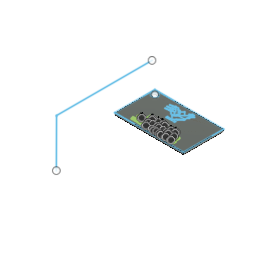
RilievoBianco_Sotto v3 (Autodesk Fusion 360 design; units mm, degrees)
Autodesk Fusion 360 part; units mm, degrees
(part 1 of 3)
sketch "Schizzo1" plane through (0, 0, 0) normal (0, 0, 1) x (1, 0, 0)
  line L0 (29.9889, 19.8901) -> (35.7373, 25.5017)
  line L1 (35.7373, 25.5017) -> (35.7373, 24.6846)
  line L2 (35.7373, 24.6846) -> (32.7498, 21.7683)
  line L3 (32.7498, 21.7683) -> (31.9129, 21.7684)
  line L4 (29.9889, 19.8901) -> (27.2751, 22.7249)
  line L5 (27.2751, 22.7249) -> (35.7303, 31.137)
  line L6 (35.7303, 31.137) -> (35.7373, 25.5017)
  line L7 (38.3163, 31.1397) -> (33.9148, 31.1342)
  line L8 (33.9148, 31.1342) -> (35.384, 32.596)
  line L9 (35.384, 32.596) -> (37.5408, 30.4282)
  line L10 (36.195, 31.7809) -> (36.8338, 32.4164)
  line L11 (36.8338, 32.4164) -> (36.8347, 31.1379)
  line L12 (38.3163, 31.1397) -> (35.7333, 28.7697)
  line L13 (36.8653, 29.8084) -> (36.8653, 28.1654)
  line L14 (36.8653, 28.1654) -> (35.7353, 27.1286)
  line L15 (32.8059, 28.2274) -> (30.0244, 31.0231)
  line L16 (30.0244, 31.0231) -> (27.8739, 28.8836)
  line L17 (27.8739, 28.8836) -> (26.8333, 29.9295)
  line L18 (26.8333, 29.9295) -> (25.5405, 29.9295)
  line L19 (25.5405, 29.9295) -> (24.3739, 31.102)
  line L20 (24.3739, 31.102) -> (22.1284, 31.102)
  line L21 (22.1284, 31.102) -> (28.8771, 24.3187)
  line L22 (28.8276, 26.6255) -> (25.5405, 29.9295)
  line L23 (-23.3316, 55.811) -> (-23.3316, -27.624)
  line L24 (-23.3316, -27.624) -> (-22.8957, -28.0621)
  line L25 (-22.8957, -28.0621) -> (18.3372, -69.5062)
  line L26 (22.1284, 31.102) -> (18.2425, 29.9166)
  line L27 (18.2425, 29.9166) -> (23.3077, 29.9166)
  line L28 (24.493, 28.7252) -> (22.0405, 28.7252)
  line L29 (22.0405, 28.7252) -> (18.2007, 27.5303)
  line L30 (18.2007, 27.5303) -> (23.0405, 27.5303)
  line L31 (23.0405, 27.5303) -> (24.0405, 26.5295)
  line L32 (24.0405, 26.5295) -> (22.5405, 26.5295)
  line L33 (22.5405, 26.5295) -> (18.724, 25.3324)
  line L34 (18.724, 25.3324) -> (23.7268, 25.3324)
  line L35 (23.7268, 25.3324) -> (25.4894, 23.6528)
  line L36 (25.4894, 23.6528) -> (28.2078, 23.6528)
  line L37 (28.2078, 23.6528) -> (25.5181, 26.5255)
  line L38 (25.5181, 26.5255) -> (24.0405, 26.5295)
  line L39 (28.8771, 24.3187) -> (27.5884, 24.3143)
  line L40 (23.0405, 27.5303) -> (22.0405, 28.7252)
  line L41 (22.5405, 26.5295) -> (23.7268, 25.3324)
  line L42 (30.085, 25.5204) -> (35.7373, 25.5017)
  line L43 (26.1075, 19.8901) -> (33.1934, 19.8901)
  line L44 (28.8276, 26.6255) -> (28.8771, 24.3187)
  line L45 (27.8739, 28.8836) -> (29.3875, 27.3623)
  line L46 (29.3875, 27.3623) -> (29.3875, 24.8264)
  line L47 (28.8566, 25.2771) -> (29.3875, 24.8264)
  line L48 (0, 34.9842) -> (60, 34.9842)
  line L49 (60, 34.9842) -> (60, -0.0158)
  line L50 (60, -0.0158) -> (0, -0.0158)
  line L51 (0, -0.0158) -> (0, 34.9842)
  line L52 (26.1075, 18.8901) -> (33.1934, 18.8901)
  line L53 (33.1934, 19.8901) -> (33.1934, 18.8901)
  line L54 (26.1075, 18.8901) -> (26.1075, 19.8901)
  line L55 (17.8462, 10.5) -> (17.8462, 13)
  line L56 (17.8462, 13) -> (18.3441, 13)
  line L57 (18.3441, 13) -> (18.9359, 11.2299)
  spline S0 degree 2 poles (18.9359, 11.2299) (19.0177, 10.9826) (19.0553, 10.8598) knots 0 0 0 1 1 1
  spline S1 degree 2 poles (19.0553, 10.8598) (19.0979, 10.9962) (19.1883, 11.2606) knots 0 0 0 1 1 1
  line L58 (19.1883, 11.2606) -> (19.7868, 13)
  line L59 (19.7868, 13) -> (20.2319, 13)
  line L60 (20.2319, 13) -> (20.2319, 10.5)
  line L61 (20.2319, 10.5) -> (19.913, 10.5)
  line L62 (19.913, 10.5) -> (19.913, 12.5924)
  line L63 (19.913, 12.5924) -> (19.1866, 10.5)
  line L64 (19.1866, 10.5) -> (18.8881, 10.5)
  line L65 (18.8881, 10.5) -> (18.1651, 12.6282)
  line L66 (18.1651, 12.6282) -> (18.1651, 10.5)
  line L67 (18.1651, 10.5) -> (17.8462, 10.5)
  spline S2 degree 2 poles (20.6122, 11.4055) (20.6122, 11.9086) (20.8919, 12.1508) knots 0 0 0 1 1 1
  spline S3 degree 2 poles (20.8919, 12.1508) (21.1255, 12.352) (21.4615, 12.352) knots 0 0 0 1 1 1
  spline S4 degree 2 poles (21.4615, 12.352) (21.8349, 12.352) (22.072, 12.1073) knots 0 0 0 1 1 1
  spline S5 degree 2 poles (22.072, 12.1073) (22.309, 11.8626) (22.309, 11.4311) knots 0 0 0 1 1 1
  spline S6 degree 2 poles (22.309, 11.4311) (22.309, 11.0815) (22.2041, 10.8811) knots 0 0 0 1 1 1
  spline S7 degree 2 poles (22.2041, 10.8811) (22.0993, 10.6808) (21.8989, 10.5699) knots 0 0 0 1 1 1
  spline S8 degree 2 poles (21.8989, 10.5699) (21.6985, 10.4591) (21.4615, 10.4591) knots 0 0 0 1 1 1
  spline S9 degree 2 poles (21.4615, 10.4591) (21.0812, 10.4591) (20.8467, 10.7029) knots 0 0 0 1 1 1
  spline S10 degree 2 poles (20.8467, 10.7029) (20.6122, 10.9468) (20.6122, 11.4055) knots 0 0 0 1 1 1
  spline S11 degree 2 poles (20.9277, 11.4055) (20.9277, 11.0576) (21.0795, 10.8845) knots 0 0 0 1 1 1
  spline S12 degree 2 poles (21.0795, 10.8845) (21.2312, 10.7115) (21.4615, 10.7115) knots 0 0 0 1 1 1
  spline S13 degree 2 poles (21.4615, 10.7115) (21.69, 10.7115) (21.8417, 10.8854) knots 0 0 0 1 1 1
  spline S14 degree 2 poles (21.8417, 10.8854) (21.9935, 11.0593) (21.9935, 11.4158) knots 0 0 0 1 1 1
  spline S15 degree 2 poles (21.9935, 11.4158) (21.9935, 11.7517) (21.8409, 11.9248) knots 0 0 0 1 1 1
  spline S16 degree 2 poles (21.8409, 11.9248) (21.6883, 12.0979) (21.4615, 12.0979) knots 0 0 0 1 1 1
  spline S17 degree 2 poles (21.4615, 12.0979) (21.2312, 12.0979) (21.0795, 11.9256) knots 0 0 0 1 1 1
  spline S18 degree 2 poles (21.0795, 11.9256) (20.9277, 11.7534) (20.9277, 11.4055) knots 0 0 0 1 1 1
  line L68 (22.6688, 10.5) -> (22.6688, 12.3111)
  line L69 (22.6688, 12.3111) -> (22.9451, 12.3111)
  line L70 (22.9451, 12.3111) -> (22.9451, 12.0535)
  spline S19 degree 2 poles (22.9451, 12.0535) (23.1446, 12.352) (23.5215, 12.352) knots 0 0 0 1 1 1
  spline S20 degree 2 poles (23.5215, 12.352) (23.6852, 12.352) (23.8225, 12.2931) knots 0 0 0 1 1 1
  spline S21 degree 2 poles (23.8225, 12.2931) (23.9598, 12.2343) (24.028, 12.1388) knots 0 0 0 1 1 1
  spline S22 degree 2 poles (24.028, 12.1388) (24.0962, 12.0433) (24.1235, 11.912) knots 0 0 0 1 1 1
  spline S23 degree 2 poles (24.1235, 11.912) (24.1405, 11.8267) (24.1405, 11.6136) knots 0 0 0 1 1 1
  line L71 (24.1405, 11.6136) -> (24.1405, 10.5)
  line L72 (24.1405, 10.5) -> (23.8336, 10.5)
  line L73 (23.8336, 10.5) -> (23.8336, 11.6016)
  spline S24 degree 2 poles (23.8336, 11.6016) (23.8336, 11.7892) (23.7977, 11.8822) knots 0 0 0 1 1 1
  spline S25 degree 2 poles (23.7977, 11.8822) (23.7619, 11.9751) (23.6707, 12.0305) knots 0 0 0 1 1 1
  spline S26 degree 2 poles (23.6707, 12.0305) (23.5795, 12.0859) (23.4567, 12.0859) knots 0 0 0 1 1 1
  spline S27 degree 2 poles (23.4567, 12.0859) (23.2606, 12.0859) (23.1182, 11.9615) knots 0 0 0 1 1 1
  spline S28 degree 2 poles (23.1182, 11.9615) (22.9758, 11.837) (22.9758, 11.4891) knots 0 0 0 1 1 1
  line L74 (22.9758, 11.4891) -> (22.9758, 10.5)
  line L75 (22.9758, 10.5) -> (22.6688, 10.5)
  line L76 (25.2814, 10.7746) -> (25.3257, 10.5034)
  spline S29 degree 2 poles (25.3257, 10.5034) (25.1961, 10.4761) (25.0938, 10.4761) knots 0 0 0 1 1 1
  spline S30 degree 2 poles (25.0938, 10.4761) (24.9267, 10.4761) (24.8346, 10.529) knots 0 0 0 1 1 1
  spline S31 degree 2 poles (24.8346, 10.529) (24.7425, 10.5819) (24.705, 10.668) knots 0 0 0 1 1 1
  spline S32 degree 2 poles (24.705, 10.668) (24.6675, 10.7541) (24.6675, 11.0304) knots 0 0 0 1 1 1
  line L77 (24.6675, 11.0304) -> (24.6675, 12.0723)
  line L78 (24.6675, 12.0723) -> (24.4424, 12.0723)
  line L79 (24.4424, 12.0723) -> (24.4424, 12.3111)
  line L80 (24.4424, 12.3111) -> (24.6675, 12.3111)
  line L81 (24.6675, 12.3111) -> (24.6675, 12.7595)
  line L82 (24.6675, 12.7595) -> (24.9727, 12.9437)
  line L83 (24.9727, 12.9437) -> (24.9727, 12.3111)
  line L84 (24.9727, 12.3111) -> (25.2814, 12.3111)
  line L85 (25.2814, 12.3111) -> (25.2814, 12.0723)
  line L86 (25.2814, 12.0723) -> (24.9727, 12.0723)
  line L87 (24.9727, 12.0723) -> (24.9727, 11.0133)
  spline S33 degree 2 poles (24.9727, 11.0133) (24.9727, 10.882) (24.9889, 10.8445) knots 0 0 0 1 1 1
  spline S34 degree 2 poles (24.9889, 10.8445) (25.0051, 10.807) (25.0418, 10.7848) knots 0 0 0 1 1 1
  spline S35 degree 2 poles (25.0418, 10.7848) (25.0784, 10.7626) (25.1467, 10.7626) knots 0 0 0 1 1 1
  spline S36 degree 2 poles (25.1467, 10.7626) (25.1978, 10.7626) (25.2814, 10.7746) knots 0 0 0 1 1 1
  line L88 (26.8213, 11.0832) -> (27.1385, 11.044)
  spline S37 degree 2 poles (27.1385, 11.044) (27.0634, 10.766) (26.8605, 10.6126) knots 0 0 0 1 1 1
  spline S38 degree 2 poles (26.8605, 10.6126) (26.6576, 10.4591) (26.3421, 10.4591) knots 0 0 0 1 1 1
  spline S39 degree 2 poles (26.3421, 10.4591) (25.9447, 10.4591) (25.712, 10.7038) knots 0 0 0 1 1 1
  spline S40 degree 2 poles (25.712, 10.7038) (25.4792, 10.9485) (25.4792, 11.3902) knots 0 0 0 1 1 1
  spline S41 degree 2 poles (25.4792, 11.3902) (25.4792, 11.8472) (25.7145, 12.0996) knots 0 0 0 1 1 1
  spline S42 degree 2 poles (25.7145, 12.0996) (25.9499, 12.352) (26.325, 12.352) knots 0 0 0 1 1 1
  spline S43 degree 2 poles (26.325, 12.352) (26.6883, 12.352) (26.9185, 12.1047) knots 0 0 0 1 1 1
  spline S44 degree 2 poles (26.9185, 12.1047) (27.1487, 11.8574) (27.1487, 11.4089) knots 0 0 0 1 1 1
  spline S45 degree 2 poles (27.1487, 11.4089) (27.1487, 11.3817) (27.147, 11.3271) knots 0 0 0 1 1 1
  line L89 (27.147, 11.3271) -> (25.7964, 11.3271)
  spline S46 degree 2 poles (25.7964, 11.3271) (25.8134, 11.0286) (25.9652, 10.8701) knots 0 0 0 1 1 1
  spline S47 degree 2 poles (25.9652, 10.8701) (26.117, 10.7115) (26.3438, 10.7115) knots 0 0 0 1 1 1
  spline S48 degree 2 poles (26.3438, 10.7115) (26.5126, 10.7115) (26.632, 10.8001) knots 0 0 0 1 1 1
  spline S49 degree 2 poles (26.632, 10.8001) (26.7514, 10.8888) (26.8213, 11.0832) knots 0 0 0 1 1 1
  line L90 (25.8134, 11.5795) -> (26.8247, 11.5795)
  spline S50 degree 2 poles (26.8247, 11.5795) (26.8042, 11.808) (26.7087, 11.9222) knots 0 0 0 1 1 1
  spline S51 degree 2 poles (26.7087, 11.9222) (26.5621, 12.0996) (26.3284, 12.0996) knots 0 0 0 1 1 1
  spline S52 degree 2 poles (26.3284, 12.0996) (26.117, 12.0996) (25.9729, 11.958) knots 0 0 0 1 1 1
  spline S53 degree 2 poles (25.9729, 11.958) (25.8288, 11.8165) (25.8134, 11.5795) knots 0 0 0 1 1 1
  line L91 (28.5334, 10.5) -> (28.5334, 13)
  line L92 (28.5334, 13) -> (29.3946, 13)
  spline S54 degree 2 poles (29.3946, 13) (29.6862, 13) (29.8397, 12.9642) knots 0 0 0 1 1 1
  spline S55 degree 2 poles (29.8397, 12.9642) (30.0546, 12.9147) (30.2063, 12.7851) knots 0 0 0 1 1 1
  spline S56 degree 2 poles (30.2063, 12.7851) (30.4042, 12.618) (30.5022, 12.3579) knots 0 0 0 1 1 1
  spline S57 degree 2 poles (30.5022, 12.3579) (30.6003, 12.0979) (30.6003, 11.7636) knots 0 0 0 1 1 1
  spline S58 degree 2 poles (30.6003, 11.7636) (30.6003, 11.4789) (30.5338, 11.2589) knots 0 0 0 1 1 1
  spline S59 degree 2 poles (30.5338, 11.2589) (30.4673, 11.0389) (30.3632, 10.8948) knots 0 0 0 1 1 1
  spline S60 degree 2 poles (30.3632, 10.8948) (30.2592, 10.7507) (30.1356, 10.668) knots 0 0 0 1 1 1
  spline S61 degree 2 poles (30.1356, 10.668) (30.0119, 10.5853) (29.8371, 10.5426) knots 0 0 0 1 1 1
  spline S62 degree 2 poles (29.8371, 10.5426) (29.6623, 10.5) (29.4355, 10.5) knots 0 0 0 1 1 1
  line L93 (29.4355, 10.5) -> (28.5334, 10.5)
  line L94 (28.8643, 10.795) -> (29.398, 10.795)
  spline S63 degree 2 poles (29.398, 10.795) (29.6453, 10.795) (29.786, 10.8411) knots 0 0 0 1 1 1
  spline S64 degree 2 poles (29.786, 10.8411) (29.9267, 10.8871) (30.0102, 10.9707) knots 0 0 0 1 1 1
  spline S65 degree 2 poles (30.0102, 10.9707) (30.1279, 11.0883) (30.1936, 11.287) knots 0 0 0 1 1 1
  spline S66 degree 2 poles (30.1936, 11.287) (30.2592, 11.4857) (30.2592, 11.7688) knots 0 0 0 1 1 1
  spline S67 degree 2 poles (30.2592, 11.7688) (30.2592, 12.161) (30.1305, 12.3716) knots 0 0 0 1 1 1
  spline S68 degree 2 poles (30.1305, 12.3716) (30.0017, 12.5822) (29.8175, 12.6538) knots 0 0 0 1 1 1
  spline S69 degree 2 poles (29.8175, 12.6538) (29.6845, 12.705) (29.3895, 12.705) knots 0 0 0 1 1 1
  line L95 (29.3895, 12.705) -> (28.8643, 12.705)
  line L96 (28.8643, 12.705) -> (28.8643, 10.795)
  line L97 (32.2561, 11.0832) -> (32.5733, 11.044)
  spline S70 degree 2 poles (32.5733, 11.044) (32.4983, 10.766) (32.2954, 10.6126) knots 0 0 0 1 1 1
  spline S71 degree 2 poles (32.2954, 10.6126) (32.0924, 10.4591) (31.7769, 10.4591) knots 0 0 0 1 1 1
  spline S72 degree 2 poles (31.7769, 10.4591) (31.3796, 10.4591) (31.1468, 10.7038) knots 0 0 0 1 1 1
  spline S73 degree 2 poles (31.1468, 10.7038) (30.9141, 10.9485) (30.9141, 11.3902) knots 0 0 0 1 1 1
  spline S74 degree 2 poles (30.9141, 11.3902) (30.9141, 11.8472) (31.1494, 12.0996) knots 0 0 0 1 1 1
  spline S75 degree 2 poles (31.1494, 12.0996) (31.3847, 12.352) (31.7599, 12.352) knots 0 0 0 1 1 1
  spline S76 degree 2 poles (31.7599, 12.352) (32.1231, 12.352) (32.3533, 12.1047) knots 0 0 0 1 1 1
  spline S77 degree 2 poles (32.3533, 12.1047) (32.5836, 11.8574) (32.5836, 11.4089) knots 0 0 0 1 1 1
  spline S78 degree 2 poles (32.5836, 11.4089) (32.5836, 11.3817) (32.5819, 11.3271) knots 0 0 0 1 1 1
  line L98 (32.5819, 11.3271) -> (31.2312, 11.3271)
  spline S79 degree 2 poles (31.2312, 11.3271) (31.2483, 11.0286) (31.4001, 10.8701) knots 0 0 0 1 1 1
  spline S80 degree 2 poles (31.4001, 10.8701) (31.5518, 10.7115) (31.7786, 10.7115) knots 0 0 0 1 1 1
  spline S81 degree 2 poles (31.7786, 10.7115) (31.9475, 10.7115) (32.0668, 10.8001) knots 0 0 0 1 1 1
  spline S82 degree 2 poles (32.0668, 10.8001) (32.1862, 10.8888) (32.2561, 11.0832) knots 0 0 0 1 1 1
  line L99 (31.2483, 11.5795) -> (32.2595, 11.5795)
  spline S83 degree 2 poles (32.2595, 11.5795) (32.2391, 11.808) (32.1436, 11.9222) knots 0 0 0 1 1 1
  spline S84 degree 2 poles (32.1436, 11.9222) (31.9969, 12.0996) (31.7633, 12.0996) knots 0 0 0 1 1 1
  spline S85 degree 2 poles (31.7633, 12.0996) (31.5518, 12.0996) (31.4077, 11.958) knots 0 0 0 1 1 1
  spline S86 degree 2 poles (31.4077, 11.958) (31.2636, 11.8165) (31.2483, 11.5795) knots 0 0 0 1 1 1
  line L100 (32.9519, 10.5) -> (32.9519, 13)
  line L101 (32.9519, 13) -> (33.2589, 13)
  line L102 (33.2589, 13) -> (33.2589, 10.5)
  line L103 (33.2589, 10.5) -> (32.9519, 10.5)
  line L104 (35.9141, 11.4806) -> (35.9141, 11.7739)
  line L105 (35.9141, 11.7739) -> (36.9731, 11.7756)
  line L106 (36.9731, 11.7756) -> (36.9731, 10.8479)
  spline S87 degree 2 poles (36.9731, 10.8479) (36.7292, 10.6535) (36.47, 10.5554) knots 0 0 0 1 1 1
  spline S88 degree 2 poles (36.47, 10.5554) (36.2108, 10.4574) (35.9379, 10.4574) knots 0 0 0 1 1 1
  spline S89 degree 2 poles (35.9379, 10.4574) (35.5696, 10.4574) (35.2686, 10.6151) knots 0 0 0 1 1 1
  spline S90 degree 2 poles (35.2686, 10.6151) (34.9676, 10.7729) (34.8141, 11.0713) knots 0 0 0 1 1 1
  spline S91 degree 2 poles (34.8141, 11.0713) (34.6606, 11.3697) (34.6606, 11.7381) knots 0 0 0 1 1 1
  spline S92 degree 2 poles (34.6606, 11.7381) (34.6606, 12.103) (34.8133, 12.4193) knots 0 0 0 1 1 1
  spline S93 degree 2 poles (34.8133, 12.4193) (34.9659, 12.7357) (35.2524, 12.8892) knots 0 0 0 1 1 1
  spline S94 degree 2 poles (35.2524, 12.8892) (35.5389, 13.0426) (35.9123, 13.0426) knots 0 0 0 1 1 1
  spline S95 degree 2 poles (35.9123, 13.0426) (36.1835, 13.0426) (36.4026, 12.9548) knots 0 0 0 1 1 1
  spline S96 degree 2 poles (36.4026, 12.9548) (36.6218, 12.867) (36.7462, 12.7101) knots 0 0 0 1 1 1
  spline S97 degree 2 poles (36.7462, 12.7101) (36.8707, 12.5532) (36.9355, 12.3008) knots 0 0 0 1 1 1
  line L107 (36.9355, 12.3008) -> (36.6371, 12.219)
  spline S98 degree 2 poles (36.6371, 12.219) (36.5808, 12.41) (36.4973, 12.5191) knots 0 0 0 1 1 1
  spline S99 degree 2 poles (36.4973, 12.5191) (36.4137, 12.6282) (36.2585, 12.6939) knots 0 0 0 1 1 1
  spline S100 degree 2 poles (36.2585, 12.6939) (36.1033, 12.7595) (35.9141, 12.7595) knots 0 0 0 1 1 1
  spline S101 degree 2 poles (35.9141, 12.7595) (35.6872, 12.7595) (35.5218, 12.6905) knots 0 0 0 1 1 1
  spline S102 degree 2 poles (35.5218, 12.6905) (35.3564, 12.6214) (35.2549, 12.5089) knots 0 0 0 1 1 1
  spline S103 degree 2 poles (35.2549, 12.5089) (35.1535, 12.3963) (35.0972, 12.2616) knots 0 0 0 1 1 1
  spline S104 degree 2 poles (35.0972, 12.2616) (35.0017, 12.0297) (35.0017, 11.7585) knots 0 0 0 1 1 1
  spline S105 degree 2 poles (35.0017, 11.7585) (35.0017, 11.4243) (35.1168, 11.1992) knots 0 0 0 1 1 1
  spline S106 degree 2 poles (35.1168, 11.1992) (35.2319, 10.9741) (35.4519, 10.8649) knots 0 0 0 1 1 1
  spline S107 degree 2 poles (35.4519, 10.8649) (35.6719, 10.7558) (35.9192, 10.7558) knots 0 0 0 1 1 1
  spline S108 degree 2 poles (35.9192, 10.7558) (36.134, 10.7558) (36.3387, 10.8385) knots 0 0 0 1 1 1
  spline S109 degree 2 poles (36.3387, 10.8385) (36.5433, 10.9212) (36.649, 11.015) knots 0 0 0 1 1 1
  line L108 (36.649, 11.015) -> (36.649, 11.4806)
  line L109 (36.649, 11.4806) -> (35.9141, 11.4806)
  spline S110 degree 2 poles (38.6033, 10.7234) (38.4328, 10.5784) (38.2751, 10.5188) knots 0 0 0 1 1 1
  spline S111 degree 2 poles (38.2751, 10.5188) (38.1173, 10.4591) (37.9366, 10.4591) knots 0 0 0 1 1 1
  spline S112 degree 2 poles (37.9366, 10.4591) (37.6381, 10.4591) (37.4778, 10.6049) knots 0 0 0 1 1 1
  spline S113 degree 2 poles (37.4778, 10.6049) (37.3175, 10.7507) (37.3175, 10.9775) knots 0 0 0 1 1 1
  spline S114 degree 2 poles (37.3175, 10.9775) (37.3175, 11.1105) (37.3781, 11.2205) knots 0 0 0 1 1 1
  spline S115 degree 2 poles (37.3781, 11.2205) (37.4386, 11.3305) (37.5367, 11.397) knots 0 0 0 1 1 1
  spline S116 degree 2 poles (37.5367, 11.397) (37.6347, 11.4635) (37.7575, 11.4976) knots 0 0 0 1 1 1
  spline S117 degree 2 poles (37.7575, 11.4976) (37.8479, 11.5215) (38.0304, 11.5437) knots 0 0 0 1 1 1
  spline S118 degree 2 poles (38.0304, 11.5437) (38.4021, 11.588) (38.5778, 11.6494) knots 0 0 0 1 1 1
  spline S119 degree 2 poles (38.5778, 11.6494) (38.5795, 11.7125) (38.5795, 11.7295) knots 0 0 0 1 1 1
  spline S120 degree 2 poles (38.5795, 11.7295) (38.5795, 11.9171) (38.4925, 11.9939) knots 0 0 0 1 1 1
  spline S121 degree 2 poles (38.4925, 11.9939) (38.3748, 12.0979) (38.1429, 12.0979) knots 0 0 0 1 1 1
  spline S122 degree 2 poles (38.1429, 12.0979) (37.9263, 12.0979) (37.8232, 12.022) knots 0 0 0 1 1 1
  spline S123 degree 2 poles (37.8232, 12.022) (37.72, 11.9461) (37.6705, 11.7534) knots 0 0 0 1 1 1
  line L110 (37.6705, 11.7534) -> (37.3704, 11.7943)
  spline S124 degree 2 poles (37.3704, 11.7943) (37.4113, 11.987) (37.5051, 12.1056) knots 0 0 0 1 1 1
  spline S125 degree 2 poles (37.5051, 12.1056) (37.5989, 12.2241) (37.7763, 12.288) knots 0 0 0 1 1 1
  spline S126 degree 2 poles (37.7763, 12.288) (37.9536, 12.352) (38.1872, 12.352) knots 0 0 0 1 1 1
  spline S127 degree 2 poles (38.1872, 12.352) (38.4192, 12.352) (38.5641, 12.2974) knots 0 0 0 1 1 1
  spline S128 degree 2 poles (38.5641, 12.2974) (38.7091, 12.2428) (38.7773, 12.1601) knots 0 0 0 1 1 1
  spline S129 degree 2 poles (38.7773, 12.1601) (38.8455, 12.0774) (38.8728, 11.9512) knots 0 0 0 1 1 1
  spline S130 degree 2 poles (38.8728, 11.9512) (38.8881, 11.8728) (38.8881, 11.6681) knots 0 0 0 1 1 1
  line L111 (38.8881, 11.6681) -> (38.8881, 11.2589)
  spline S131 degree 2 poles (38.8881, 11.2589) (38.8881, 10.8308) (38.9077, 10.7174) knots 0 0 0 1 1 1
  spline S132 degree 2 poles (38.9077, 10.7174) (38.9274, 10.604) (38.9853, 10.5) knots 0 0 0 1 1 1
  line L112 (38.9853, 10.5) -> (38.6647, 10.5)
  spline S133 degree 2 poles (38.6647, 10.5) (38.617, 10.5955) (38.6033, 10.7234) knots 0 0 0 1 1 1
  spline S134 degree 2 poles (38.5778, 11.4089) (38.4106, 11.3407) (38.0764, 11.293) knots 0 0 0 1 1 1
  spline S135 degree 2 poles (38.0764, 11.293) (37.8871, 11.2657) (37.8087, 11.2316) knots 0 0 0 1 1 1
  spline S136 degree 2 poles (37.8087, 11.2316) (37.7302, 11.1975) (37.6876, 11.1318) knots 0 0 0 1 1 1
  spline S137 degree 2 poles (37.6876, 11.1318) (37.645, 11.0662) (37.645, 10.986) knots 0 0 0 1 1 1
  spline S138 degree 2 poles (37.645, 10.986) (37.645, 10.8632) (37.7379, 10.7814) knots 0 0 0 1 1 1
  spline S139 degree 2 poles (37.7379, 10.7814) (37.8308, 10.6995) (38.0099, 10.6995) knots 0 0 0 1 1 1
  spline S140 degree 2 poles (38.0099, 10.6995) (38.1872, 10.6995) (38.3254, 10.7771) knots 0 0 0 1 1 1
  spline S141 degree 2 poles (38.3254, 10.7771) (38.4635, 10.8547) (38.5283, 10.9894) knots 0 0 0 1 1 1
  spline S142 degree 2 poles (38.5283, 10.9894) (38.5778, 11.0935) (38.5778, 11.2964) knots 0 0 0 1 1 1
  line L113 (38.5778, 11.2964) -> (38.5778, 11.4089)
  line L114 (39.3571, 10.5) -> (39.3571, 13)
  line L115 (39.3571, 13) -> (39.6641, 13)
  line L116 (39.6641, 13) -> (39.6641, 10.5)
  line L117 (39.6641, 10.5) -> (39.3571, 10.5)
  line L118 (40.133, 10.5) -> (40.133, 13)
  line L119 (40.133, 13) -> (40.44, 13)
  line L120 (40.44, 13) -> (40.44, 10.5)
  line L121 (40.44, 10.5) -> (40.133, 10.5)
  spline S143 degree 2 poles (40.8015, 11.4055) (40.8015, 11.9086) (41.0812, 12.1508) knots 0 0 0 1 1 1
  spline S144 degree 2 poles (41.0812, 12.1508) (41.3148, 12.352) (41.6507, 12.352) knots 0 0 0 1 1 1
  spline S145 degree 2 poles (41.6507, 12.352) (42.0242, 12.352) (42.2613, 12.1073) knots 0 0 0 1 1 1
  spline S146 degree 2 poles (42.2613, 12.1073) (42.4983, 11.8626) (42.4983, 11.4311) knots 0 0 0 1 1 1
  spline S147 degree 2 poles (42.4983, 11.4311) (42.4983, 11.0815) (42.3934, 10.8811) knots 0 0 0 1 1 1
  spline S148 degree 2 poles (42.3934, 10.8811) (42.2885, 10.6808) (42.0882, 10.5699) knots 0 0 0 1 1 1
  spline S149 degree 2 poles (42.0882, 10.5699) (41.8878, 10.4591) (41.6507, 10.4591) knots 0 0 0 1 1 1
  spline S150 degree 2 poles (41.6507, 10.4591) (41.2705, 10.4591) (41.036, 10.7029) knots 0 0 0 1 1 1
  spline S151 degree 2 poles (41.036, 10.7029) (40.8015, 10.9468) (40.8015, 11.4055) knots 0 0 0 1 1 1
  spline S152 degree 2 poles (41.117, 11.4055) (41.117, 11.0576) (41.2688, 10.8845) knots 0 0 0 1 1 1
  spline S153 degree 2 poles (41.2688, 10.8845) (41.4205, 10.7115) (41.6507, 10.7115) knots 0 0 0 1 1 1
  spline S154 degree 2 poles (41.6507, 10.7115) (41.8793, 10.7115) (42.031, 10.8854) knots 0 0 0 1 1 1
  spline S155 degree 2 poles (42.031, 10.8854) (42.1828, 11.0593) (42.1828, 11.4158) knots 0 0 0 1 1 1
  spline S156 degree 2 poles (42.1828, 11.4158) (42.1828, 11.7517) (42.0302, 11.9248) knots 0 0 0 1 1 1
  spline S157 degree 2 poles (42.0302, 11.9248) (41.8776, 12.0979) (41.6507, 12.0979) knots 0 0 0 1 1 1
  spline S158 degree 2 poles (41.6507, 12.0979) (41.4205, 12.0979) (41.2688, 11.9256) knots 0 0 0 1 1 1
  spline S159 degree 2 poles (41.2688, 11.9256) (41.117, 11.7534) (41.117, 11.4055) knots 0 0 0 1 1 1
  line L122 (12.5989, 7.4014) -> (12.911, 7.4287)
  spline S160 degree 2 poles (12.911, 7.4287) (12.9332, 7.2411) (13.0142, 7.1209) knots 0 0 0 1 1 1
  spline S161 degree 2 poles (13.0142, 7.1209) (13.0952, 7.0007) (13.2657, 6.9265) knots 0 0 0 1 1 1
  spline S162 degree 2 poles (13.2657, 6.9265) (13.4362, 6.8523) (13.6494, 6.8523) knots 0 0 0 1 1 1
  spline S163 degree 2 poles (13.6494, 6.8523) (13.8387, 6.8523) (13.9836, 6.9086) knots 0 0 0 1 1 1
  spline S164 degree 2 poles (13.9836, 6.9086) (14.1286, 6.9649) (14.1994, 7.0629) knots 0 0 0 1 1 1
  spline S165 degree 2 poles (14.1994, 7.0629) (14.2701, 7.161) (14.2701, 7.2769) knots 0 0 0 1 1 1
  spline S166 degree 2 poles (14.2701, 7.2769) (14.2701, 7.3946) (14.2019, 7.4824) knots 0 0 0 1 1 1
  spline S167 degree 2 poles (14.2019, 7.4824) (14.1337, 7.5703) (13.9768, 7.6299) knots 0 0 0 1 1 1
  spline S168 degree 2 poles (13.9768, 7.6299) (13.8762, 7.6692) (13.5317, 7.7519) knots 0 0 0 1 1 1
  spline S169 degree 2 poles (13.5317, 7.7519) (13.1872, 7.8346) (13.0491, 7.9079) knots 0 0 0 1 1 1
  spline S170 degree 2 poles (13.0491, 7.9079) (12.8701, 8.0017) (12.7822, 8.1407) knots 0 0 0 1 1 1
  spline S171 degree 2 poles (12.7822, 8.1407) (12.6944, 8.2797) (12.6944, 8.4519) knots 0 0 0 1 1 1
  spline S172 degree 2 poles (12.6944, 8.4519) (12.6944, 8.6412) (12.8018, 8.8058) knots 0 0 0 1 1 1
  spline S173 degree 2 poles (12.8018, 8.8058) (12.9093, 8.9703) (13.1156, 9.0556) knots 0 0 0 1 1 1
  spline S174 degree 2 poles (13.1156, 9.0556) (13.322, 9.1409) (13.5744, 9.1409) knots 0 0 0 1 1 1
  spline S175 degree 2 poles (13.5744, 9.1409) (13.8523, 9.1409) (14.0646, 9.0513) knots 0 0 0 1 1 1
  spline S176 degree 2 poles (14.0646, 9.0513) (14.2769, 8.9618) (14.3912, 8.7879) knots 0 0 0 1 1 1
  spline S177 degree 2 poles (14.3912, 8.7879) (14.5055, 8.6139) (14.514, 8.3939) knots 0 0 0 1 1 1
  line L123 (14.514, 8.3939) -> (14.1968, 8.3701)
  spline S178 degree 2 poles (14.1968, 8.3701) (14.1712, 8.6071) (14.0237, 8.7282) knots 0 0 0 1 1 1
  spline S179 degree 2 poles (14.0237, 8.7282) (13.8762, 8.8492) (13.588, 8.8492) knots 0 0 0 1 1 1
  spline S180 degree 2 poles (13.588, 8.8492) (13.2879, 8.8492) (13.1506, 8.7393) knots 0 0 0 1 1 1
  spline S181 degree 2 poles (13.1506, 8.7393) (13.0133, 8.6293) (13.0133, 8.4741) knots 0 0 0 1 1 1
  spline S182 degree 2 poles (13.0133, 8.4741) (13.0133, 8.3394) (13.1105, 8.2524) knots 0 0 0 1 1 1
  spline S183 degree 2 poles (13.1105, 8.2524) (13.206, 8.1654) (13.6093, 8.0742) knots 0 0 0 1 1 1
  spline S184 degree 2 poles (13.6093, 8.0742) (14.0126, 7.9829) (14.1627, 7.9147) knots 0 0 0 1 1 1
  spline S185 degree 2 poles (14.1627, 7.9147) (14.381, 7.8141) (14.485, 7.6598) knots 0 0 0 1 1 1
  spline S186 degree 2 poles (14.485, 7.6598) (14.589, 7.5055) (14.589, 7.3042) knots 0 0 0 1 1 1
  spline S187 degree 2 poles (14.589, 7.3042) (14.589, 7.1047) (14.4748, 6.9282) knots 0 0 0 1 1 1
  spline S188 degree 2 poles (14.4748, 6.9282) (14.3605, 6.7517) (14.1465, 6.6536) knots 0 0 0 1 1 1
  spline S189 degree 2 poles (14.1465, 6.6536) (13.9325, 6.5556) (13.6647, 6.5556) knots 0 0 0 1 1 1
  spline S190 degree 2 poles (13.6647, 6.5556) (13.3254, 6.5556) (13.096, 6.6545) knots 0 0 0 1 1 1
  spline S191 degree 2 poles (13.096, 6.6545) (12.8666, 6.7534) (12.7362, 6.9521) knots 0 0 0 1 1 1
  spline S192 degree 2 poles (12.7362, 6.9521) (12.6057, 7.1508) (12.5989, 7.4014) knots 0 0 0 1 1 1
  spline S193 degree 2 poles (14.8874, 7.5038) (14.8874, 8.0068) (15.1671, 8.249) knots 0 0 0 1 1 1
  spline S194 degree 2 poles (15.1671, 8.249) (15.4008, 8.4502) (15.7367, 8.4502) knots 0 0 0 1 1 1
  spline S195 degree 2 poles (15.7367, 8.4502) (16.1102, 8.4502) (16.3472, 8.2055) knots 0 0 0 1 1 1
  spline S196 degree 2 poles (16.3472, 8.2055) (16.5842, 7.9608) (16.5842, 7.5293) knots 0 0 0 1 1 1
  spline S197 degree 2 poles (16.5842, 7.5293) (16.5842, 7.1797) (16.4794, 6.9794) knots 0 0 0 1 1 1
  spline S198 degree 2 poles (16.4794, 6.9794) (16.3745, 6.779) (16.1741, 6.6681) knots 0 0 0 1 1 1
  spline S199 degree 2 poles (16.1741, 6.6681) (15.9737, 6.5573) (15.7367, 6.5573) knots 0 0 0 1 1 1
  spline S200 degree 2 poles (15.7367, 6.5573) (15.3564, 6.5573) (15.1219, 6.8012) knots 0 0 0 1 1 1
  spline S201 degree 2 poles (15.1219, 6.8012) (14.8874, 7.045) (14.8874, 7.5038) knots 0 0 0 1 1 1
  spline S202 degree 2 poles (15.2029, 7.5038) (15.2029, 7.1559) (15.3547, 6.9828) knots 0 0 0 1 1 1
  spline S203 degree 2 poles (15.3547, 6.9828) (15.5065, 6.8097) (15.7367, 6.8097) knots 0 0 0 1 1 1
  spline S204 degree 2 poles (15.7367, 6.8097) (15.9652, 6.8097) (16.117, 6.9836) knots 0 0 0 1 1 1
  spline S205 degree 2 poles (16.117, 6.9836) (16.2688, 7.1576) (16.2688, 7.514) knots 0 0 0 1 1 1
  spline S206 degree 2 poles (16.2688, 7.514) (16.2688, 7.8499) (16.1161, 8.023) knots 0 0 0 1 1 1
  spline S207 degree 2 poles (16.1161, 8.023) (15.9635, 8.1961) (15.7367, 8.1961) knots 0 0 0 1 1 1
  spline S208 degree 2 poles (15.7367, 8.1961) (15.5065, 8.1961) (15.3547, 8.0239) knots 0 0 0 1 1 1
  spline S209 degree 2 poles (15.3547, 8.0239) (15.2029, 7.8516) (15.2029, 7.5038) knots 0 0 0 1 1 1
  line L124 (17.0174, 6.5982) -> (17.0174, 8.1705)
  line L125 (17.0174, 8.1705) -> (16.7462, 8.1705)
  line L126 (16.7462, 8.1705) -> (16.7462, 8.4093)
  line L127 (16.7462, 8.4093) -> (17.0174, 8.4093)
  line L128 (17.0174, 8.4093) -> (17.0174, 8.602)
  spline S210 degree 2 poles (17.0174, 8.602) (17.0174, 8.7844) (17.0498, 8.8731) knots 0 0 0 1 1 1
  spline S211 degree 2 poles (17.0498, 8.8731) (17.0941, 8.9925) (17.2058, 9.0667) knots 0 0 0 1 1 1
  spline S212 degree 2 poles (17.2058, 9.0667) (17.3175, 9.1409) (17.5188, 9.1409) knots 0 0 0 1 1 1
  spline S213 degree 2 poles (17.5188, 9.1409) (17.6484, 9.1409) (17.8053, 9.1102) knots 0 0 0 1 1 1
  line L129 (17.8053, 9.1102) -> (17.7592, 8.8424)
  spline S214 degree 2 poles (17.7592, 8.8424) (17.6637, 8.8595) (17.5784, 8.8595) knots 0 0 0 1 1 1
  spline S215 degree 2 poles (17.5784, 8.8595) (17.4386, 8.8595) (17.3806, 8.7998) knots 0 0 0 1 1 1
  spline S216 degree 2 poles (17.3806, 8.7998) (17.3226, 8.7401) (17.3226, 8.5764) knots 0 0 0 1 1 1
  line L130 (17.3226, 8.5764) -> (17.3226, 8.4093)
  line L131 (17.3226, 8.4093) -> (17.6756, 8.4093)
  line L132 (17.6756, 8.4093) -> (17.6756, 8.1705)
  line L133 (17.6756, 8.1705) -> (17.3226, 8.1705)
  line L134 (17.3226, 8.1705) -> (17.3226, 6.5982)
  line L135 (17.3226, 6.5982) -> (17.0174, 6.5982)
  line L136 (18.5846, 6.8728) -> (18.6289, 6.6016)
  spline S217 degree 2 poles (18.6289, 6.6016) (18.4993, 6.5744) (18.397, 6.5744) knots 0 0 0 1 1 1
  spline S218 degree 2 poles (18.397, 6.5744) (18.2299, 6.5744) (18.1378, 6.6272) knots 0 0 0 1 1 1
  spline S219 degree 2 poles (18.1378, 6.6272) (18.0457, 6.6801) (18.0082, 6.7662) knots 0 0 0 1 1 1
  spline S220 degree 2 poles (18.0082, 6.7662) (17.9707, 6.8523) (17.9707, 7.1286) knots 0 0 0 1 1 1
  line L137 (17.9707, 7.1286) -> (17.9707, 8.1705)
  line L138 (17.9707, 8.1705) -> (17.7456, 8.1705)
  line L139 (17.7456, 8.1705) -> (17.7456, 8.4093)
  line L140 (17.7456, 8.4093) -> (17.9707, 8.4093)
  line L141 (17.9707, 8.4093) -> (17.9707, 8.8578)
  line L142 (17.9707, 8.8578) -> (18.2759, 9.042)
  line L143 (18.2759, 9.042) -> (18.2759, 8.4093)
  line L144 (18.2759, 8.4093) -> (18.5846, 8.4093)
  line L145 (18.5846, 8.4093) -> (18.5846, 8.1705)
  line L146 (18.5846, 8.1705) -> (18.2759, 8.1705)
  line L147 (18.2759, 8.1705) -> (18.2759, 7.1115)
  spline S221 degree 2 poles (18.2759, 7.1115) (18.2759, 6.9802) (18.2921, 6.9427) knots 0 0 0 1 1 1
  spline S222 degree 2 poles (18.2921, 6.9427) (18.3083, 6.9052) (18.345, 6.883) knots 0 0 0 1 1 1
  spline S223 degree 2 poles (18.345, 6.883) (18.3817, 6.8608) (18.4499, 6.8608) knots 0 0 0 1 1 1
  spline S224 degree 2 poles (18.4499, 6.8608) (18.501, 6.8608) (18.5846, 6.8728) knots 0 0 0 1 1 1
  line L148 (19.219, 6.5982) -> (18.6647, 8.4093)
  line L149 (18.6647, 8.4093) -> (18.9819, 8.4093)
  line L150 (18.9819, 8.4093) -> (19.2701, 7.3639)
  line L151 (19.2701, 7.3639) -> (19.3776, 6.9751)
  spline S225 degree 2 poles (19.3776, 6.9751) (19.3844, 7.0041) (19.4714, 7.3486) knots 0 0 0 1 1 1
  line L152 (19.4714, 7.3486) -> (19.7595, 8.4093)
  line L153 (19.7595, 8.4093) -> (20.075, 8.4093)
  line L154 (20.075, 8.4093) -> (20.3462, 7.3588)
  line L155 (20.3462, 7.3588) -> (20.4366, 7.0126)
  line L156 (20.4366, 7.0126) -> (20.5406, 7.3622)
  line L157 (20.5406, 7.3622) -> (20.851, 8.4093)
  line L158 (20.851, 8.4093) -> (21.1494, 8.4093)
  line L159 (21.1494, 8.4093) -> (20.5832, 6.5982)
  line L160 (20.5832, 6.5982) -> (20.2643, 6.5982)
  line L161 (20.2643, 6.5982) -> (19.9761, 7.6828)
  line L162 (19.9761, 7.6828) -> (19.9062, 7.9915)
  line L163 (19.9062, 7.9915) -> (19.5396, 6.5982)
  line L164 (19.5396, 6.5982) -> (19.219, 6.5982)
  spline S226 degree 2 poles (22.5887, 6.8216) (22.4181, 6.6767) (22.2604, 6.617) knots 0 0 0 1 1 1
  spline S227 degree 2 poles (22.2604, 6.617) (22.1027, 6.5573) (21.9219, 6.5573) knots 0 0 0 1 1 1
  spline S228 degree 2 poles (21.9219, 6.5573) (21.6235, 6.5573) (21.4632, 6.7031) knots 0 0 0 1 1 1
  spline S229 degree 2 poles (21.4632, 6.7031) (21.3029, 6.8489) (21.3029, 7.0757) knots 0 0 0 1 1 1
  spline S230 degree 2 poles (21.3029, 7.0757) (21.3029, 7.2087) (21.3634, 7.3187) knots 0 0 0 1 1 1
  spline S231 degree 2 poles (21.3634, 7.3187) (21.4239, 7.4287) (21.522, 7.4952) knots 0 0 0 1 1 1
  spline S232 degree 2 poles (21.522, 7.4952) (21.6201, 7.5617) (21.7428, 7.5958) knots 0 0 0 1 1 1
  spline S233 degree 2 poles (21.7428, 7.5958) (21.8332, 7.6197) (22.0157, 7.6419) knots 0 0 0 1 1 1
  spline S234 degree 2 poles (22.0157, 7.6419) (22.3874, 7.6862) (22.5631, 7.7476) knots 0 0 0 1 1 1
  spline S235 degree 2 poles (22.5631, 7.7476) (22.5648, 7.8107) (22.5648, 7.8278) knots 0 0 0 1 1 1
  spline S236 degree 2 poles (22.5648, 7.8278) (22.5648, 8.0153) (22.4778, 8.0921) knots 0 0 0 1 1 1
  spline S237 degree 2 poles (22.4778, 8.0921) (22.3602, 8.1961) (22.1282, 8.1961) knots 0 0 0 1 1 1
  spline S238 degree 2 poles (22.1282, 8.1961) (21.9117, 8.1961) (21.8085, 8.1202) knots 0 0 0 1 1 1
  spline S239 degree 2 poles (21.8085, 8.1202) (21.7053, 8.0443) (21.6559, 7.8516) knots 0 0 0 1 1 1
  line L165 (21.6559, 7.8516) -> (21.3557, 7.8926)
  spline S240 degree 2 poles (21.3557, 7.8926) (21.3967, 8.0853) (21.4905, 8.2038) knots 0 0 0 1 1 1
  spline S241 degree 2 poles (21.4905, 8.2038) (21.5842, 8.3223) (21.7616, 8.3863) knots 0 0 0 1 1 1
  spline S242 degree 2 poles (21.7616, 8.3863) (21.9389, 8.4502) (22.1726, 8.4502) knots 0 0 0 1 1 1
  spline S243 degree 2 poles (22.1726, 8.4502) (22.4045, 8.4502) (22.5495, 8.3956) knots 0 0 0 1 1 1
  spline S244 degree 2 poles (22.5495, 8.3956) (22.6944, 8.3411) (22.7626, 8.2584) knots 0 0 0 1 1 1
  spline S245 degree 2 poles (22.7626, 8.2584) (22.8308, 8.1756) (22.8581, 8.0495) knots 0 0 0 1 1 1
  spline S246 degree 2 poles (22.8581, 8.0495) (22.8735, 7.971) (22.8735, 7.7664) knots 0 0 0 1 1 1
  line L166 (22.8735, 7.7664) -> (22.8735, 7.3571)
  spline S247 degree 2 poles (22.8735, 7.3571) (22.8735, 6.9291) (22.8931, 6.8157) knots 0 0 0 1 1 1
  spline S248 degree 2 poles (22.8931, 6.8157) (22.9127, 6.7023) (22.9707, 6.5982) knots 0 0 0 1 1 1
  line L167 (22.9707, 6.5982) -> (22.6501, 6.5982)
  spline S249 degree 2 poles (22.6501, 6.5982) (22.6023, 6.6937) (22.5887, 6.8216) knots 0 0 0 1 1 1
  spline S250 degree 2 poles (22.5631, 7.5072) (22.396, 7.4389) (22.0617, 7.3912) knots 0 0 0 1 1 1
  spline S251 degree 2 poles (22.0617, 7.3912) (21.8724, 7.3639) (21.794, 7.3298) knots 0 0 0 1 1 1
  spline S252 degree 2 poles (21.794, 7.3298) (21.7156, 7.2957) (21.6729, 7.23) knots 0 0 0 1 1 1
  spline S253 degree 2 poles (21.6729, 7.23) (21.6303, 7.1644) (21.6303, 7.0842) knots 0 0 0 1 1 1
  spline S254 degree 2 poles (21.6303, 7.0842) (21.6303, 6.9615) (21.7232, 6.8796) knots 0 0 0 1 1 1
  spline S255 degree 2 poles (21.7232, 6.8796) (21.8162, 6.7977) (21.9952, 6.7977) knots 0 0 0 1 1 1
  spline S256 degree 2 poles (21.9952, 6.7977) (22.1726, 6.7977) (22.3107, 6.8753) knots 0 0 0 1 1 1
  spline S257 degree 2 poles (22.3107, 6.8753) (22.4488, 6.9529) (22.5136, 7.0877) knots 0 0 0 1 1 1
  spline S258 degree 2 poles (22.5136, 7.0877) (22.5631, 7.1917) (22.5631, 7.3946) knots 0 0 0 1 1 1
  line L168 (22.5631, 7.3946) -> (22.5631, 7.5072)
  line L169 (23.3458, 6.5982) -> (23.3458, 8.4093)
  line L170 (23.3458, 8.4093) -> (23.6221, 8.4093)
  line L171 (23.6221, 8.4093) -> (23.6221, 8.1347)
  spline S259 degree 2 poles (23.6221, 8.1347) (23.7278, 8.3274) (23.8174, 8.3888) knots 0 0 0 1 1 1
  spline S260 degree 2 poles (23.8174, 8.3888) (23.9069, 8.4502) (24.0143, 8.4502) knots 0 0 0 1 1 1
  spline S261 degree 2 poles (24.0143, 8.4502) (24.1695, 8.4502) (24.3298, 8.3513) knots 0 0 0 1 1 1
  line L172 (24.3298, 8.3513) -> (24.2241, 8.0665)
  spline S262 degree 2 poles (24.2241, 8.0665) (24.1115, 8.133) (23.999, 8.133) knots 0 0 0 1 1 1
  spline S263 degree 2 poles (23.999, 8.133) (23.8984, 8.133) (23.8182, 8.0725) knots 0 0 0 1 1 1
  spline S264 degree 2 poles (23.8182, 8.0725) (23.7381, 8.0119) (23.704, 7.9045) knots 0 0 0 1 1 1
  spline S265 degree 2 poles (23.704, 7.9045) (23.6528, 7.7408) (23.6528, 7.5464) knots 0 0 0 1 1 1
  line L173 (23.6528, 7.5464) -> (23.6528, 6.5982)
  line L174 (23.6528, 6.5982) -> (23.3458, 6.5982)
  line L175 (25.752, 7.1814) -> (26.0692, 7.1422)
  spline S266 degree 2 poles (26.0692, 7.1422) (25.9942, 6.8643) (25.7913, 6.7108) knots 0 0 0 1 1 1
  spline S267 degree 2 poles (25.7913, 6.7108) (25.5883, 6.5573) (25.2728, 6.5573) knots 0 0 0 1 1 1
  spline S268 degree 2 poles (25.2728, 6.5573) (24.8755, 6.5573) (24.6427, 6.802) knots 0 0 0 1 1 1
  spline S269 degree 2 poles (24.6427, 6.802) (24.41, 7.0467) (24.41, 7.4884) knots 0 0 0 1 1 1
  spline S270 degree 2 poles (24.41, 7.4884) (24.41, 7.9454) (24.6453, 8.1978) knots 0 0 0 1 1 1
  spline S271 degree 2 poles (24.6453, 8.1978) (24.8806, 8.4502) (25.2558, 8.4502) knots 0 0 0 1 1 1
  spline S272 degree 2 poles (25.2558, 8.4502) (25.619, 8.4502) (25.8492, 8.2029) knots 0 0 0 1 1 1
  spline S273 degree 2 poles (25.8492, 8.2029) (26.0795, 7.9557) (26.0795, 7.5072) knots 0 0 0 1 1 1
  spline S274 degree 2 poles (26.0795, 7.5072) (26.0795, 7.4799) (26.0778, 7.4253) knots 0 0 0 1 1 1
  line L176 (26.0778, 7.4253) -> (24.7271, 7.4253)
  spline S275 degree 2 poles (24.7271, 7.4253) (24.7442, 7.1269) (24.896, 6.9683) knots 0 0 0 1 1 1
  spline S276 degree 2 poles (24.896, 6.9683) (25.0477, 6.8097) (25.2746, 6.8097) knots 0 0 0 1 1 1
  spline S277 degree 2 poles (25.2746, 6.8097) (25.4434, 6.8097) (25.5628, 6.8984) knots 0 0 0 1 1 1
  spline S278 degree 2 poles (25.5628, 6.8984) (25.6821, 6.987) (25.752, 7.1814) knots 0 0 0 1 1 1
  line L177 (24.7442, 7.6777) -> (25.7555, 7.6777)
  spline S279 degree 2 poles (25.7555, 7.6777) (25.735, 7.9062) (25.6395, 8.0205) knots 0 0 0 1 1 1
  spline S280 degree 2 poles (25.6395, 8.0205) (25.4928, 8.1978) (25.2592, 8.1978) knots 0 0 0 1 1 1
  spline S281 degree 2 poles (25.2592, 8.1978) (25.0477, 8.1978) (24.9036, 8.0563) knots 0 0 0 1 1 1
  spline S282 degree 2 poles (24.9036, 8.0563) (24.7595, 7.9147) (24.7442, 7.6777) knots 0 0 0 1 1 1
  line L178 (27.4642, 6.5982) -> (27.4642, 9.0982)
  line L179 (27.4642, 9.0982) -> (28.3254, 9.0982)
  spline S283 degree 2 poles (28.3254, 9.0982) (28.617, 9.0982) (28.7705, 9.0624) knots 0 0 0 1 1 1
  spline S284 degree 2 poles (28.7705, 9.0624) (28.9853, 9.013) (29.1371, 8.8834) knots 0 0 0 1 1 1
  spline S285 degree 2 poles (29.1371, 8.8834) (29.3349, 8.7162) (29.433, 8.4562) knots 0 0 0 1 1 1
  spline S286 degree 2 poles (29.433, 8.4562) (29.531, 8.1961) (29.531, 7.8619) knots 0 0 0 1 1 1
  spline S287 degree 2 poles (29.531, 7.8619) (29.531, 7.5771) (29.4645, 7.3571) knots 0 0 0 1 1 1
  spline S288 degree 2 poles (29.4645, 7.3571) (29.398, 7.1371) (29.294, 6.993) knots 0 0 0 1 1 1
  spline S289 degree 2 poles (29.294, 6.993) (29.19, 6.8489) (29.0663, 6.7662) knots 0 0 0 1 1 1
  spline S290 degree 2 poles (29.0663, 6.7662) (28.9427, 6.6835) (28.7679, 6.6409) knots 0 0 0 1 1 1
  spline S291 degree 2 poles (28.7679, 6.6409) (28.5931, 6.5982) (28.3663, 6.5982) knots 0 0 0 1 1 1
  line L180 (28.3663, 6.5982) -> (27.4642, 6.5982)
  line L181 (27.795, 6.8932) -> (28.3288, 6.8932)
  spline S292 degree 2 poles (28.3288, 6.8932) (28.5761, 6.8932) (28.7167, 6.9393) knots 0 0 0 1 1 1
  spline S293 degree 2 poles (28.7167, 6.9393) (28.8574, 6.9853) (28.941, 7.0689) knots 0 0 0 1 1 1
  spline S294 degree 2 poles (28.941, 7.0689) (29.0587, 7.1866) (29.1243, 7.3852) knots 0 0 0 1 1 1
  spline S295 degree 2 poles (29.1243, 7.3852) (29.19, 7.5839) (29.19, 7.867) knots 0 0 0 1 1 1
  spline S296 degree 2 poles (29.19, 7.867) (29.19, 8.2592) (29.0612, 8.4698) knots 0 0 0 1 1 1
  spline S297 degree 2 poles (29.0612, 8.4698) (28.9325, 8.6804) (28.7483, 8.752) knots 0 0 0 1 1 1
  spline S298 degree 2 poles (28.7483, 8.752) (28.6153, 8.8032) (28.3203, 8.8032) knots 0 0 0 1 1 1
  line L182 (28.3203, 8.8032) -> (27.795, 8.8032)
  line L183 (27.795, 8.8032) -> (27.795, 6.8932)
  line L184 (31.1869, 7.1814) -> (31.5041, 7.1422)
  spline S299 degree 2 poles (31.5041, 7.1422) (31.4291, 6.8643) (31.2261, 6.7108) knots 0 0 0 1 1 1
  spline S300 degree 2 poles (31.2261, 6.7108) (31.0232, 6.5573) (30.7077, 6.5573) knots 0 0 0 1 1 1
  spline S301 degree 2 poles (30.7077, 6.5573) (30.3104, 6.5573) (30.0776, 6.802) knots 0 0 0 1 1 1
  spline S302 degree 2 poles (30.0776, 6.802) (29.8448, 7.0467) (29.8448, 7.4884) knots 0 0 0 1 1 1
  spline S303 degree 2 poles (29.8448, 7.4884) (29.8448, 7.9454) (30.0802, 8.1978) knots 0 0 0 1 1 1
  spline S304 degree 2 poles (30.0802, 8.1978) (30.3155, 8.4502) (30.6907, 8.4502) knots 0 0 0 1 1 1
  spline S305 degree 2 poles (30.6907, 8.4502) (31.0539, 8.4502) (31.2841, 8.2029) knots 0 0 0 1 1 1
  spline S306 degree 2 poles (31.2841, 8.2029) (31.5143, 7.9557) (31.5143, 7.5072) knots 0 0 0 1 1 1
  spline S307 degree 2 poles (31.5143, 7.5072) (31.5143, 7.4799) (31.5126, 7.4253) knots 0 0 0 1 1 1
  line L185 (31.5126, 7.4253) -> (30.162, 7.4253)
  spline S308 degree 2 poles (30.162, 7.4253) (30.1791, 7.1269) (30.3308, 6.9683) knots 0 0 0 1 1 1
  spline S309 degree 2 poles (30.3308, 6.9683) (30.4826, 6.8097) (30.7094, 6.8097) knots 0 0 0 1 1 1
  spline S310 degree 2 poles (30.7094, 6.8097) (30.8782, 6.8097) (30.9976, 6.8984) knots 0 0 0 1 1 1
  spline S311 degree 2 poles (30.9976, 6.8984) (31.117, 6.987) (31.1869, 7.1814) knots 0 0 0 1 1 1
  line L186 (30.1791, 7.6777) -> (31.1903, 7.6777)
  spline S312 degree 2 poles (31.1903, 7.6777) (31.1698, 7.9062) (31.0744, 8.0205) knots 0 0 0 1 1 1
  spline S313 degree 2 poles (31.0744, 8.0205) (30.9277, 8.1978) (30.6941, 8.1978) knots 0 0 0 1 1 1
  spline S314 degree 2 poles (30.6941, 8.1978) (30.4826, 8.1978) (30.3385, 8.0563) knots 0 0 0 1 1 1
  spline S315 degree 2 poles (30.3385, 8.0563) (30.1944, 7.9147) (30.1791, 7.6777) knots 0 0 0 1 1 1
  line L187 (32.3926, 6.5982) -> (31.7036, 8.4093)
  line L188 (31.7036, 8.4093) -> (32.0276, 8.4093)
  line L189 (32.0276, 8.4093) -> (32.4164, 7.3247)
  spline S316 degree 2 poles (32.4164, 7.3247) (32.4795, 7.149) (32.5324, 6.9598) knots 0 0 0 1 1 1
  spline S317 degree 2 poles (32.5324, 6.9598) (32.5733, 7.103) (32.6467, 7.3042) knots 0 0 0 1 1 1
  line L190 (32.6467, 7.3042) -> (33.0491, 8.4093)
  line L191 (33.0491, 8.4093) -> (33.3646, 8.4093)
  line L192 (33.3646, 8.4093) -> (32.6791, 6.5982)
  line L193 (32.6791, 6.5982) -> (32.3926, 6.5982)
  line L194 (34.8755, 7.1814) -> (35.1927, 7.1422)
  spline S318 degree 2 poles (35.1927, 7.1422) (35.1177, 6.8643) (34.9147, 6.7108) knots 0 0 0 1 1 1
  spline S319 degree 2 poles (34.9147, 6.7108) (34.7118, 6.5573) (34.3963, 6.5573) knots 0 0 0 1 1 1
  spline S320 degree 2 poles (34.3963, 6.5573) (33.999, 6.5573) (33.7662, 6.802) knots 0 0 0 1 1 1
  spline S321 degree 2 poles (33.7662, 6.802) (33.5334, 7.0467) (33.5334, 7.4884) knots 0 0 0 1 1 1
  spline S322 degree 2 poles (33.5334, 7.4884) (33.5334, 7.9454) (33.7688, 8.1978) knots 0 0 0 1 1 1
  spline S323 degree 2 poles (33.7688, 8.1978) (34.0041, 8.4502) (34.3793, 8.4502) knots 0 0 0 1 1 1
  spline S324 degree 2 poles (34.3793, 8.4502) (34.7425, 8.4502) (34.9727, 8.2029) knots 0 0 0 1 1 1
  spline S325 degree 2 poles (34.9727, 8.2029) (35.2029, 7.9557) (35.2029, 7.5072) knots 0 0 0 1 1 1
  spline S326 degree 2 poles (35.2029, 7.5072) (35.2029, 7.4799) (35.2012, 7.4253) knots 0 0 0 1 1 1
  line L195 (35.2012, 7.4253) -> (33.8506, 7.4253)
  spline S327 degree 2 poles (33.8506, 7.4253) (33.8677, 7.1269) (34.0194, 6.9683) knots 0 0 0 1 1 1
  spline S328 degree 2 poles (34.0194, 6.9683) (34.1712, 6.8097) (34.398, 6.8097) knots 0 0 0 1 1 1
  spline S329 degree 2 poles (34.398, 6.8097) (34.5669, 6.8097) (34.6862, 6.8984) knots 0 0 0 1 1 1
  spline S330 degree 2 poles (34.6862, 6.8984) (34.8056, 6.987) (34.8755, 7.1814) knots 0 0 0 1 1 1
  line L196 (33.8677, 7.6777) -> (34.8789, 7.6777)
  spline S331 degree 2 poles (34.8789, 7.6777) (34.8585, 7.9062) (34.763, 8.0205) knots 0 0 0 1 1 1
  spline S332 degree 2 poles (34.763, 8.0205) (34.6163, 8.1978) (34.3827, 8.1978) knots 0 0 0 1 1 1
  spline S333 degree 2 poles (34.3827, 8.1978) (34.1712, 8.1978) (34.0271, 8.0563) knots 0 0 0 1 1 1
  spline S334 degree 2 poles (34.0271, 8.0563) (33.883, 7.9147) (33.8677, 7.6777) knots 0 0 0 1 1 1
  line L197 (35.5713, 6.5982) -> (35.5713, 9.0982)
  line L198 (35.5713, 9.0982) -> (35.8782, 9.0982)
  line L199 (35.8782, 9.0982) -> (35.8782, 6.5982)
  line L200 (35.8782, 6.5982) -> (35.5713, 6.5982)
  spline S335 degree 2 poles (36.2398, 7.5038) (36.2398, 8.0068) (36.5194, 8.249) knots 0 0 0 1 1 1
  spline S336 degree 2 poles (36.5194, 8.249) (36.7531, 8.4502) (37.089, 8.4502) knots 0 0 0 1 1 1
  spline S337 degree 2 poles (37.089, 8.4502) (37.4625, 8.4502) (37.6995, 8.2055) knots 0 0 0 1 1 1
  spline S338 degree 2 poles (37.6995, 8.2055) (37.9366, 7.9608) (37.9366, 7.5293) knots 0 0 0 1 1 1
  spline S339 degree 2 poles (37.9366, 7.5293) (37.9366, 7.1797) (37.8317, 6.9794) knots 0 0 0 1 1 1
  spline S340 degree 2 poles (37.8317, 6.9794) (37.7268, 6.779) (37.5264, 6.6681) knots 0 0 0 1 1 1
  spline S341 degree 2 poles (37.5264, 6.6681) (37.3261, 6.5573) (37.089, 6.5573) knots 0 0 0 1 1 1
  spline S342 degree 2 poles (37.089, 6.5573) (36.7087, 6.5573) (36.4743, 6.8012) knots 0 0 0 1 1 1
  spline S343 degree 2 poles (36.4743, 6.8012) (36.2398, 7.045) (36.2398, 7.5038) knots 0 0 0 1 1 1
  spline S344 degree 2 poles (36.5553, 7.5038) (36.5553, 7.1559) (36.707, 6.9828) knots 0 0 0 1 1 1
  spline S345 degree 2 poles (36.707, 6.9828) (36.8588, 6.8097) (37.089, 6.8097) knots 0 0 0 1 1 1
  spline S346 degree 2 poles (37.089, 6.8097) (37.3175, 6.8097) (37.4693, 6.9836) knots 0 0 0 1 1 1
  spline S347 degree 2 poles (37.4693, 6.9836) (37.6211, 7.1576) (37.6211, 7.514) knots 0 0 0 1 1 1
  spline S348 degree 2 poles (37.6211, 7.514) (37.6211, 7.8499) (37.4685, 8.023) knots 0 0 0 1 1 1
  spline S349 degree 2 poles (37.4685, 8.023) (37.3158, 8.1961) (37.089, 8.1961) knots 0 0 0 1 1 1
  spline S350 degree 2 poles (37.089, 8.1961) (36.8588, 8.1961) (36.707, 8.0239) knots 0 0 0 1 1 1
  spline S351 degree 2 poles (36.707, 8.0239) (36.5553, 7.8516) (36.5553, 7.5038) knots 0 0 0 1 1 1
  line L201 (38.2964, 5.9042) -> (38.2964, 8.4093)
  line L202 (38.2964, 8.4093) -> (38.5761, 8.4093)
  line L203 (38.5761, 8.4093) -> (38.5761, 8.1739)
  spline S352 degree 2 poles (38.5761, 8.1739) (38.675, 8.3121) (38.7995, 8.3811) knots 0 0 0 1 1 1
  spline S353 degree 2 poles (38.7995, 8.3811) (38.9239, 8.4502) (39.1013, 8.4502) knots 0 0 0 1 1 1
  spline S354 degree 2 poles (39.1013, 8.4502) (39.3332, 8.4502) (39.5106, 8.3308) knots 0 0 0 1 1 1
  spline S355 degree 2 poles (39.5106, 8.3308) (39.6879, 8.2115) (39.7783, 7.994) knots 0 0 0 1 1 1
  spline S356 degree 2 poles (39.7783, 7.994) (39.8687, 7.7766) (39.8687, 7.5174) knots 0 0 0 1 1 1
  spline S357 degree 2 poles (39.8687, 7.5174) (39.8687, 7.2394) (39.7689, 7.0169) knots 0 0 0 1 1 1
  spline S358 degree 2 poles (39.7689, 7.0169) (39.6692, 6.7943) (39.479, 6.6758) knots 0 0 0 1 1 1
  spline S359 degree 2 poles (39.479, 6.6758) (39.2889, 6.5573) (39.0791, 6.5573) knots 0 0 0 1 1 1
  spline S360 degree 2 poles (39.0791, 6.5573) (38.9256, 6.5573) (38.8037, 6.6221) knots 0 0 0 1 1 1
  spline S361 degree 2 poles (38.8037, 6.6221) (38.6818, 6.6869) (38.6033, 6.7858) knots 0 0 0 1 1 1
  line L204 (38.6033, 6.7858) -> (38.6033, 5.9042)
  line L205 (38.6033, 5.9042) -> (38.2964, 5.9042)
  spline S362 degree 2 poles (38.5744, 7.4935) (38.5744, 7.1439) (38.7159, 6.9768) knots 0 0 0 1 1 1
  spline S363 degree 2 poles (38.7159, 6.9768) (38.8574, 6.8097) (39.0587, 6.8097) knots 0 0 0 1 1 1
  spline S364 degree 2 poles (39.0587, 6.8097) (39.2633, 6.8097) (39.4091, 6.9828) knots 0 0 0 1 1 1
  spline S365 degree 2 poles (39.4091, 6.9828) (39.5549, 7.1559) (39.5549, 7.5191) knots 0 0 0 1 1 1
  spline S366 degree 2 poles (39.5549, 7.5191) (39.5549, 7.8653) (39.4125, 8.0375) knots 0 0 0 1 1 1
  spline S367 degree 2 poles (39.4125, 8.0375) (39.2701, 8.2098) (39.0723, 8.2098) knots 0 0 0 1 1 1
  spline S368 degree 2 poles (39.0723, 8.2098) (38.8762, 8.2098) (38.7253, 8.0264) knots 0 0 0 1 1 1
  spline S369 degree 2 poles (38.7253, 8.0264) (38.5744, 7.8431) (38.5744, 7.4935) knots 0 0 0 1 1 1
  line L206 (40.2387, 6.5982) -> (40.2387, 8.4093)
  line L207 (40.2387, 8.4093) -> (40.5133, 8.4093)
  line L208 (40.5133, 8.4093) -> (40.5133, 8.1552)
  spline S370 degree 2 poles (40.5133, 8.1552) (40.5986, 8.2882) (40.7401, 8.3692) knots 0 0 0 1 1 1
  spline S371 degree 2 poles (40.7401, 8.3692) (40.8816, 8.4502) (41.0624, 8.4502) knots 0 0 0 1 1 1
  spline S372 degree 2 poles (41.0624, 8.4502) (41.2636, 8.4502) (41.3924, 8.3666) knots 0 0 0 1 1 1
  spline S373 degree 2 poles (41.3924, 8.3666) (41.5211, 8.2831) (41.574, 8.133) knots 0 0 0 1 1 1
  spline S374 degree 2 poles (41.574, 8.133) (41.7889, 8.4502) (42.1334, 8.4502) knots 0 0 0 1 1 1
  spline S375 degree 2 poles (42.1334, 8.4502) (42.4028, 8.4502) (42.5477, 8.301) knots 0 0 0 1 1 1
  spline S376 degree 2 poles (42.5477, 8.301) (42.6927, 8.1518) (42.6927, 7.8414) knots 0 0 0 1 1 1
  line L209 (42.6927, 7.8414) -> (42.6927, 6.5982)
  line L210 (42.6927, 6.5982) -> (42.3874, 6.5982)
  line L211 (42.3874, 6.5982) -> (42.3874, 7.7391)
  spline S377 degree 2 poles (42.3874, 7.7391) (42.3874, 7.9233) (42.3576, 8.0043) knots 0 0 0 1 1 1
  spline S378 degree 2 poles (42.3576, 8.0043) (42.3278, 8.0853) (42.2493, 8.1347) knots 0 0 0 1 1 1
  spline S379 degree 2 poles (42.2493, 8.1347) (42.1709, 8.1842) (42.0651, 8.1842) knots 0 0 0 1 1 1
  spline S380 degree 2 poles (42.0651, 8.1842) (41.8741, 8.1842) (41.748, 8.0571) knots 0 0 0 1 1 1
  spline S381 degree 2 poles (41.748, 8.0571) (41.6218, 7.9301) (41.6218, 7.6504) knots 0 0 0 1 1 1
  line L212 (41.6218, 7.6504) -> (41.6218, 6.5982)
  line L213 (41.6218, 6.5982) -> (41.3148, 6.5982)
  line L214 (41.3148, 6.5982) -> (41.3148, 7.7749)
  spline S382 degree 2 poles (41.3148, 7.7749) (41.3148, 7.9795) (41.2398, 8.0819) knots 0 0 0 1 1 1
  spline S383 degree 2 poles (41.2398, 8.0819) (41.1647, 8.1842) (40.9942, 8.1842) knots 0 0 0 1 1 1